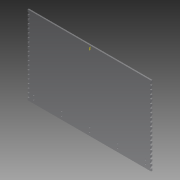
# Autodesk Inventor part: case_rear
Saved by Autodesk Inventor 2014 (Build 180170000, 170)
## iProperties
Created: 2013-08-29
Part Number: case_rear
Material: Polycarbonate, Clear
Document SubType Name: Modeling
Designer: Edward
Density: 1.2 g/cm^3
Appearance: Polycarbonate - Clear
Author: Edward
Autodesk Inventor part; units mm, degrees
ref_plane "YZ Plane" through (0, 0, 0) normal (1, 0, 0) x (0, 1, 0)
ref_plane "XZ Plane" through (0, 0, 0) normal (0, 1, 0) x (-1, 0, 0)
ref_plane "XY Plane" through (0, 0, 0) normal (0, 0, 1) x (1, 0, 0)
sketch "Sketch1" plane through (0, 0, 0) normal (0, 0, 1) x (1, 0, 0)
  line L0 (303, -45.4136) -> (309.35, -45.4136) projected
  line L1 (303, -45.4136) -> (303, -33.5636) projected
  line L2 (303, 348.2864) -> (309.35, 348.2864) projected
  line L3 (-309.35, 348.2864) -> (-303, 348.2864) projected
  line L4 (-303, -33.5636) -> (-303, -45.4136) projected
  line L5 (303, -45.4136) -> (-303, -45.4136)
  line L6 (-303, -45.4136) -> (-303, 348.2864)
  line L7 (-303, 348.2864) -> (303, 348.2864)
  line L8 (303, 348.2864) -> (303, -45.4136)
  point P0 (0, 0)
  constraints: 8 end point, 2 parallel, 1 horizontal, 1 perpendicular
extrude "Extrusion1" add sketch "Sketch1" along normal blind 6.35
sketch "Sketch3" plane through (303, -45.4136, 0) normal (1, 0, 0) x (0, 0, -1)
  line L0 (0, 393.7) -> (0, 0) projected
  line L1 (-6.35, 0) -> (-6.35, 393.7) projected
  line L2 (0, 21.85) -> (-6.35, 21.85) projected
  line L3 (0, 31.85) -> (-6.35, 31.85) projected
  point P0 (0, 45.4136)
extrude "Extrusion3" add sketch "Sketch3" along normal blind 6.35
pattern_linear "Rectangular Pattern1" count 18 spacing 20 along (0, 1, 0) of "Extrusion3"
sketch "Sketch4" plane through (303, 348.2864, 6.35) normal (1, 0, 0) x (0, 0, -1)
  line L0 (6.35, 0) -> (0, 0) projected
  line L1 (0, -21.85) -> (0, 0) projected
  circle A0 centre (454.35, -377.7) radius 2.75 projected
  circle A1 centre (259.35, -357.7) radius 2.75 projected
  circle A2 centre (64.35, -377.7) radius 2.75 projected
  circle A3 centre (64.35, -357.7) radius 2.75 projected
  circle A4 centre (259.35, -377.7) radius 2.75 projected
  circle A5 centre (454.35, -357.7) radius 2.75 projected
  arc A6 (30.35, -355.2) -> (18.35, -355.2) centre (24.35, -355.2) ccw projected
  line L2 (30.35, -355.2) -> (30.35, -380.2) projected
  arc A7 (18.35, -380.2) -> (30.35, -380.2) centre (24.35, -380.2) ccw projected
  line L3 (18.35, -380.2) -> (18.35, -355.2) projected
  arc A8 (488.35, -380.2) -> (500.35, -380.2) centre (494.35, -380.2) ccw projected
  line L4 (488.35, -380.2) -> (488.35, -355.2) projected
  arc A9 (500.35, -355.2) -> (488.35, -355.2) centre (494.35, -355.2) ccw projected
  line L5 (500.35, -355.2) -> (500.35, -380.2) projected
  line L6 (6.35, -393.7) -> (513.2999, -393.7) projected
  line L7 (513.2999, -393.7) -> (513.2999, -381.85) projected
  line L8 (513.2999, -381.85) -> (519.6499, -381.85) projected
  line L9 (519.6499, -371.85) -> (519.6499, -381.85) projected
  line L10 (513.2999, -371.85) -> (519.6499, -371.85) projected
  line L11 (513.2999, -371.85) -> (513.2999, -361.85) projected
  line L12 (513.2999, -361.85) -> (519.6499, -361.85) projected
  line L13 (519.6499, -351.85) -> (519.6499, -361.85) projected
  line L14 (513.2999, -351.85) -> (519.6499, -351.85) projected
  line L15 (513.2999, -351.85) -> (513.2999, -341.85) projected
  line L16 (513.2999, -341.85) -> (519.6499, -341.85) projected
  line L17 (519.6499, -331.85) -> (519.6499, -341.85) projected
  line L18 (513.2999, -331.85) -> (519.6499, -331.85) projected
  line L19 (513.2999, -331.85) -> (513.2999, -321.85) projected
  line L20 (513.2999, -321.85) -> (519.6499, -321.85) projected
  line L21 (519.6499, -311.85) -> (519.6499, -321.85) projected
  line L22 (513.2999, -311.85) -> (519.6499, -311.85) projected
  line L23 (513.2999, -311.85) -> (513.2999, -301.85) projected
  line L24 (513.2999, -301.85) -> (519.6499, -301.85) projected
  line L25 (519.6499, -291.85) -> (519.6499, -301.85) projected
  line L26 (513.2999, -291.85) -> (519.6499, -291.85) projected
  line L27 (513.2999, -291.85) -> (513.2999, -281.85) projected
  line L28 (513.2999, -281.85) -> (519.6499, -281.85) projected
  line L29 (519.6499, -271.85) -> (519.6499, -281.85) projected
  line L30 (513.2999, -271.85) -> (519.6499, -271.85) projected
  line L31 (513.2999, -271.85) -> (513.2999, -261.85) projected
  line L32 (513.2999, -261.85) -> (519.6499, -261.85) projected
  line L33 (519.6499, -251.85) -> (519.6499, -261.85) projected
  line L34 (513.2999, -251.85) -> (519.6499, -251.85) projected
  line L35 (513.2999, -251.85) -> (513.2999, -241.85) projected
  line L36 (513.2999, -241.85) -> (519.6499, -241.85) projected
  line L37 (519.6499, -231.85) -> (519.6499, -241.85) projected
  line L38 (513.2999, -231.85) -> (519.6499, -231.85) projected
  line L39 (513.2999, -231.85) -> (513.2999, -221.85) projected
  line L40 (513.2999, -221.85) -> (519.6499, -221.85) projected
  line L41 (519.6499, -211.85) -> (519.6499, -221.85) projected
  line L42 (513.2999, -211.85) -> (519.6499, -211.85) projected
  line L43 (513.2999, -211.85) -> (513.2999, -201.85) projected
  line L44 (513.2999, -201.85) -> (519.6499, -201.85) projected
  line L45 (519.6499, -191.85) -> (519.6499, -201.85) projected
  line L46 (513.2999, -191.85) -> (519.6499, -191.85) projected
  line L47 (513.2999, -191.85) -> (513.2999, -181.85) projected
  line L48 (513.2999, -181.85) -> (519.6499, -181.85) projected
  line L49 (519.6499, -171.85) -> (519.6499, -181.85) projected
  line L50 (513.2999, -171.85) -> (519.6499, -171.85) projected
  line L51 (513.2999, -171.85) -> (513.2999, -161.85) projected
  line L52 (513.2999, -161.85) -> (519.6499, -161.85) projected
  line L53 (519.6499, -151.85) -> (519.6499, -161.85) projected
  line L54 (513.2999, -151.85) -> (519.6499, -151.85) projected
  line L55 (513.2999, -151.85) -> (513.2999, -141.85) projected
  line L56 (513.2999, -141.85) -> (519.6499, -141.85) projected
  line L57 (519.6499, -131.85) -> (519.6499, -141.85) projected
  line L58 (513.2999, -131.85) -> (519.6499, -131.85) projected
  line L59 (513.2999, -131.85) -> (513.2999, -121.85) projected
  line L60 (513.2999, -121.85) -> (519.6499, -121.85) projected
  line L61 (519.6499, -111.85) -> (519.6499, -121.85) projected
  line L62 (513.2999, -111.85) -> (519.6499, -111.85) projected
  line L63 (513.2999, -111.85) -> (513.2999, -101.85) projected
  line L64 (513.2999, -101.85) -> (519.6499, -101.85) projected
  line L65 (519.6499, -91.85) -> (519.6499, -101.85) projected
  line L66 (513.2999, -91.85) -> (519.6499, -91.85) projected
  line L67 (513.2999, -91.85) -> (513.2999, -81.85) projected
  line L68 (513.2999, -81.85) -> (519.6499, -81.85) projected
  line L69 (519.6499, -71.85) -> (519.6499, -81.85) projected
  line L70 (513.2999, -71.85) -> (519.6499, -71.85) projected
  line L71 (513.2999, -71.85) -> (513.2999, -61.85) projected
  line L72 (513.2999, -61.85) -> (519.6499, -61.85) projected
  line L73 (519.6499, -51.85) -> (519.6499, -61.85) projected
  line L74 (513.2999, -51.85) -> (519.6499, -51.85) projected
  line L75 (513.2999, -51.85) -> (513.2999, -41.85) projected
  line L76 (513.2999, -41.85) -> (519.6499, -41.85) projected
  line L77 (519.6499, -31.85) -> (519.6499, -41.85) projected
  line L78 (513.2999, -31.85) -> (519.6499, -31.85) projected
  line L79 (513.2999, -31.85) -> (513.2999, -21.85) projected
  line L80 (513.2999, -21.85) -> (519.6499, -21.85) projected
  line L81 (519.6499, -11.85) -> (519.6499, -21.85) projected
  line L82 (513.2999, -11.85) -> (519.6499, -11.85) projected
  line L83 (513.2999, -11.85) -> (513.2999, 0) projected
  line L84 (513.2999, 0) -> (6.35, 0) projected
  line L85 (6.35, 0) -> (6.35, -11.85) projected
  line L86 (6.35, -11.85) -> (0, -11.85) projected
  line L87 (0, -21.85) -> (0, -11.85) projected
  line L88 (6.35, -21.85) -> (0, -21.85) projected
  line L89 (6.35, -21.85) -> (6.35, -31.85) projected
  line L90 (6.35, -31.85) -> (0, -31.85) projected
  line L91 (0, -41.85) -> (0, -31.85) projected
  line L92 (6.35, -41.85) -> (0, -41.85) projected
  line L93 (6.35, -41.85) -> (6.35, -51.85) projected
  line L94 (6.35, -51.85) -> (0, -51.85) projected
  line L95 (0, -61.85) -> (0, -51.85) projected
  line L96 (6.35, -61.85) -> (0, -61.85) projected
  line L97 (6.35, -61.85) -> (6.35, -71.85) projected
  line L98 (6.35, -71.85) -> (0, -71.85) projected
  line L99 (0, -81.85) -> (0, -71.85) projected
  line L100 (6.35, -81.85) -> (0, -81.85) projected
  line L101 (6.35, -81.85) -> (6.35, -91.85) projected
  line L102 (6.35, -91.85) -> (0, -91.85) projected
  line L103 (0, -101.85) -> (0, -91.85) projected
  line L104 (6.35, -101.85) -> (0, -101.85) projected
  line L105 (6.35, -101.85) -> (6.35, -111.85) projected
  line L106 (6.35, -111.85) -> (0, -111.85) projected
  line L107 (0, -121.85) -> (0, -111.85) projected
  line L108 (6.35, -121.85) -> (0, -121.85) projected
  line L109 (6.35, -121.85) -> (6.35, -131.85) projected
  line L110 (6.35, -131.85) -> (0, -131.85) projected
  line L111 (0, -141.85) -> (0, -131.85) projected
  line L112 (6.35, -141.85) -> (0, -141.85) projected
  line L113 (6.35, -141.85) -> (6.35, -151.85) projected
  line L114 (6.35, -151.85) -> (0, -151.85) projected
  line L115 (0, -161.85) -> (0, -151.85) projected
  line L116 (6.35, -161.85) -> (0, -161.85) projected
  line L117 (6.35, -161.85) -> (6.35, -171.85) projected
  line L118 (6.35, -171.85) -> (0, -171.85) projected
  line L119 (0, -181.85) -> (0, -171.85) projected
  line L120 (6.35, -181.85) -> (0, -181.85) projected
  line L121 (6.35, -181.85) -> (6.35, -191.85) projected
  line L122 (6.35, -191.85) -> (0, -191.85) projected
  line L123 (0, -201.85) -> (0, -191.85) projected
  line L124 (6.35, -201.85) -> (0, -201.85) projected
  line L125 (6.35, -201.85) -> (6.35, -211.85) projected
  line L126 (6.35, -211.85) -> (0, -211.85) projected
  line L127 (0, -221.85) -> (0, -211.85) projected
  line L128 (6.35, -221.85) -> (0, -221.85) projected
  line L129 (6.35, -221.85) -> (6.35, -231.85) projected
  line L130 (6.35, -231.85) -> (0, -231.85) projected
  line L131 (0, -241.85) -> (0, -231.85) projected
  line L132 (6.35, -241.85) -> (0, -241.85) projected
  line L133 (6.35, -241.85) -> (6.35, -251.85) projected
  line L134 (6.35, -251.85) -> (0, -251.85) projected
  line L135 (0, -261.85) -> (0, -251.85) projected
  line L136 (6.35, -261.85) -> (0, -261.85) projected
  line L137 (6.35, -261.85) -> (6.35, -271.85) projected
  line L138 (6.35, -271.85) -> (0, -271.85) projected
  line L139 (0, -281.85) -> (0, -271.85) projected
  line L140 (6.35, -281.85) -> (0, -281.85) projected
  line L141 (6.35, -281.85) -> (6.35, -291.85) projected
  line L142 (6.35, -291.85) -> (0, -291.85) projected
  line L143 (0, -301.85) -> (0, -291.85) projected
  line L144 (6.35, -301.85) -> (0, -301.85) projected
  line L145 (6.35, -301.85) -> (6.35, -311.85) projected
  line L146 (6.35, -311.85) -> (0, -311.85) projected
  line L147 (0, -321.85) -> (0, -311.85) projected
  line L148 (6.35, -321.85) -> (0, -321.85) projected
  line L149 (6.35, -321.85) -> (6.35, -331.85) projected
  line L150 (6.35, -331.85) -> (0, -331.85) projected
  line L151 (0, -341.85) -> (0, -331.85) projected
  line L152 (6.35, -341.85) -> (0, -341.85) projected
  line L153 (6.35, -341.85) -> (6.35, -351.85) projected
  line L154 (6.35, -351.85) -> (0, -351.85) projected
  line L155 (0, -361.85) -> (0, -351.85) projected
  line L156 (6.35, -361.85) -> (0, -361.85) projected
  line L157 (6.35, -361.85) -> (6.35, -371.85) projected
  line L158 (6.35, -371.85) -> (0, -371.85) projected
  line L159 (0, -381.85) -> (0, -371.85) projected
  line L160 (6.35, -381.85) -> (0, -381.85) projected
  line L161 (6.35, -381.85) -> (6.35, -393.7) projected
  line L162 (6.35, -393.7) -> (0, -393.7) projected
  line L163 (0, -393.7) -> (0, -371.85) projected
  point P0 (6.35, -348.2864)
extrude "Extrusion4" add sketch "Sketch4" along normal blind 6.35 contours L85 L86 L1 L0 | L160 L161 L162 L163
ref_plane "Work Plane1" through (0, 326.4364, 6.35) normal (1, 0, 0) x (0, 0, -1)
mirror "Mirror1" about plane through (0, 326.4364, 6.35) normal (1, 0, 0) of "Extrusion3", "Rectangular Pattern1", "Extrusion4"
sketch "Sketch6" plane through (0, 0, 6.35) normal (0, 0, 1) x (1, 0, 0)
  circle A0 centre (0, -29.4136) radius 2.75 projected
  circle A1 centre (0, -9.4136) radius 2.75 projected
  circle A2 centre (140, -29.4136) radius 2.75 projected
  circle A3 centre (140, -9.4136) radius 2.75 projected
  circle A4 centre (280, -9.4136) radius 2.75 projected
  circle A5 centre (280, -29.4136) radius 2.75 projected
  circle A6 centre (-280, -29.4136) radius 2.75 projected
  circle A7 centre (-280, -9.4136) radius 2.75 projected
  circle A8 centre (-140, -9.4136) radius 2.75 projected
  circle A9 centre (-140, -29.4136) radius 2.75 projected
  point P0 (0, 0)
extrude "Extrusion5" cut sketch "Sketch6" against normal through all
body "Solid1"
